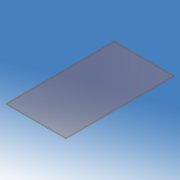
# Autodesk Inventor part: NASA-20-EBOX-LID-01
Saved by Autodesk Inventor 2020 (Build 240168000, 168)
## iProperties
Created: 2019-09-23
Part Number: NASA-20-EBOX-LID-01
Material: Polycarbonate, Smoke
Document SubType Name: Modeling
Designer: mpark
Density: 1.2 g/cm^3
Appearance: Polycarbonate - Smoked
Author: mpark
Autodesk Inventor part; units mm, degrees
ref_plane "YZ Plane" through (0, 0, 0) normal (1, 0, 0) x (0, 1, 0)
ref_plane "XZ Plane" through (0, 0, 0) normal (0, 1, 0) x (-1, 0, 0)
ref_plane "XY Plane" through (0, 0, 0) normal (0, 0, 1) x (1, 0, 0)
sketch "Sketch1" plane through (0, 0, 0) normal (0, 1, 0) x (-1, 0, 0)
  line L0 (82.55, 149.225) -> (-82.55, 149.225)
  line L1 (-82.55, 149.225) -> (-82.55, -149.225)
  line L2 (-82.55, -149.225) -> (82.55, -149.225)
  line L3 (82.55, -149.225) -> (82.55, 149.225)
  line L4 (82.55, 149.225) -> (-82.55, -149.225) construction
  line L5 (-82.55, 149.225) -> (82.55, -149.225) construction
  point P0 (0, 0)
  dimension "d0" = 165.1
  dimension "d1" = 298.45
  constraints: 12 end point, 2 midpoint, 2 parallel, 1 horizontal, 1 perpendicular
  measures "d0" distance of L2.end L1.end
  measures "d1" distance of L1.end L0.end
extrude "Extrusion1" add sketch "Sketch1" along normal blind 3.175
body "Solid1"
